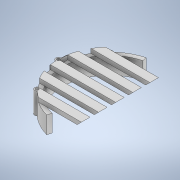
# Autodesk Inventor part: RoofNewShooterCup
Saved by Autodesk Inventor 2020 (Build 240168000, 168)
## iProperties
Created: 2021-04-22
Part Number: RoofNewShooterCup
Material: Generic
Document SubType Name: Modeling
Designer: tdmp4
Density: 1 g/cm^3
Appearance: Default
Author: tdmp4
Autodesk Inventor part; units mm, degrees
ref_plane "YZ Plane" through (0, 0, 0) normal (1, 0, 0) x (0, 1, 0)
ref_plane "XZ Plane" through (0, 0, 0) normal (0, 1, 0) x (-1, 0, 0)
ref_plane "XY Plane" through (0, 0, 0) normal (0, 0, 1) x (1, 0, 0)
sketch "Sketch1" plane through (0, 0, 0) normal (0, 1, 0) x (-1, 0, 0)
  circle A0 centre (0, 0) radius 72.39
  circle A1 centre (0, 0) radius 76.2
  circle A2 centre (76.2, 0) radius 3.81
  circle A3 centre (76.2, 0) radius 2.286
  circle A4 centre (0, 0) radius 69.85
  line L0 (0, 0) -> (53.8815, -53.8815)
  line L1 (0, 0) -> (76.2, 0) construction
  line L2 (0, 0) -> (53.8815, 53.8815)
  line L3 (0, 0) -> (76.2, 0) construction
  circle A5 centre (53.8815, 53.8815) radius 3.81
  circle A6 centre (53.8815, -53.8815) radius 3.81
  circle A7 centre (53.8815, -53.8815) radius 2.286
  circle A8 centre (53.8815, 53.8815) radius 2.286
  line L4 (0, 0) -> (18.0785, 67.4699)
  line L5 (0, 0) -> (69.85, 0) construction
  line L6 (18.0785, 67.4699) -> (19.722, 73.6035)
  line L7 (0, 0) -> (19.722, -73.6035)
  line L8 (0, 0) -> (76.2, 0) construction
  point P0 (76.1048, 3.8088)
  point P1 (56.5074, 51.1209)
  point P2 (51.1875, 51.1875)
  point P3 (49.3914, 49.3914)
  point P4 (49.3914, -49.3914)
  point P5 (51.1875, -51.1875)
  point P6 (56.5074, -51.1209)
  point P7 (76.1048, -3.8088)
  point P8 (51.1209, -56.5074)
  point P9 (18.0785, -67.4699)
  point P10 (51.1209, 56.5074)
  dimension "d4" = 139.7
  dimension "d0" = 144.78
  dimension "d1" = 152.4
  dimension "d2" = 7.62
  dimension "d3" = 4.572
  dimension "d5" = 45
  dimension "d6" = 45
  dimension "d7" = 4.572
  dimension "d8" = 4.572
  dimension "d11" = 75
  dimension "d12" = 75
  constraints: 18 end point, 8 centre point, 8 coincident, 5 point on circle, 4 equal length, 4 horizontal, 1 tangent, 3 other
  measures "d0" diameter of A0
  measures "d1" diameter of A1
  measures "d2" diameter of A2
  measures "d3" diameter of A3
  measures "d5" angle of L0 L1
  measures "d6" angle of L3 L2
  measures "d7" diameter of A7
  measures "d8" diameter of A8
  measures "d11" angle of L5 L4
  measures "d12" angle of L7 L8
extrude "Extrusion1" add sketch "Sketch1" along normal blind 25.4 contours A0 L0 A4 L2 | A2 A1 A6 A0 | A0 A5 A1 A2 | A2 A1 A3 | L2 A4 L6 A0 | A5 A1 A8 L2 | A0 L6 A1 A5 | L2 A8 A1 A5 | A6 A1 L7 A0 | A0 L7 A4 L0 | A6 A1 A7 L0 | L0 A7 A1 A6 | A2 A1 A3 | A5 A1 A8 | A6 A1 A7
sketch "Sketch2" plane through (0, 25.4, 0) normal (0, 1, 0) x (1, 0, 0)
  arc A0 (-76.1048, 3.8088) -> (-76.1048, -3.8088) centre (-76.2, 0) ccw projected
  line L0 (-80.01, 0) -> (-80.01, -76.2)
  line L1 (-80.01, -76.2) -> (-80.01, 76.2)
  line L2 (-80.01, 76.2) -> (21.59, 76.2) construction
  line L3 (-74.93, 63.5) -> (-74.93, 50.8)
  line L4 (-74.93, 50.8) -> (21.59, 50.8)
  line L5 (21.59, 50.8) -> (21.59, 38.1)
  line L6 (21.59, 38.1) -> (-74.93, 38.1)
  line L7 (-74.93, 38.1) -> (-74.93, 25.4)
  line L8 (-74.93, 25.4) -> (21.59, 25.4)
  line L9 (21.59, 25.4) -> (21.59, 12.7)
  line L10 (21.59, 12.7) -> (-74.93, 12.7)
  line L11 (-74.93, 12.7) -> (-74.93, 0)
  line L12 (-74.93, 0) -> (21.59, 0)
  line L13 (21.59, 0) -> (21.59, -12.7)
  line L14 (21.59, -12.7) -> (-74.93, -12.7)
  line L15 (-74.93, -12.7) -> (-74.93, -25.4)
  line L16 (-74.93, -25.4) -> (21.59, -25.4)
  line L17 (21.59, -25.4) -> (21.59, -38.1)
  line L18 (21.59, -38.1) -> (-74.93, -38.1)
  line L19 (-74.93, -38.1) -> (-74.93, -50.8)
  line L20 (-74.93, -50.8) -> (21.59, -50.8)
  line L21 (21.59, -50.8) -> (21.59, -63.5)
  line L22 (21.59, -63.5) -> (-75.5152, -63.5)
  line L23 (-75.5152, -63.5) -> (-75.5152, -76.2)
  line L24 (-75.5152, -76.2) -> (-80.01, -76.2)
  line L25 (-74.93, 63.5) -> (-74.93, 76.2)
  line L26 (-74.93, 63.5) -> (-80.01, 63.5)
  line L27 (-74.93, 50.8) -> (-80.01, 50.8)
  line L28 (-75.5152, -63.5) -> (-80.01, -63.5)
  circle A1 centre (-53.8815, -53.8815) radius 2.286 projected
  circle A2 centre (-53.8815, -53.8815) radius 2.286
  circle A3 centre (-53.8815, 53.8815) radius 2.286 projected
  circle A4 centre (-53.8815, 53.8815) radius 2.286
  circle A5 centre (-76.2, 0) radius 2.286 projected
  circle A6 centre (-76.2, 0) radius 2.286
  line L29 (-75.5152, -63.5) -> (-80.01, -63.5)
  point P0 (0, 0)
  point P1 (-73.914, 0)
  point P2 (-74.93, 1.9008)
  dimension "d13" = 76.2
  dimension "d14" = 152.4
  dimension "d20" = 12.7
  dimension "d21" = 12.7
  dimension "d22" = 12.7
  dimension "d23" = 12.7
  dimension "d24" = 96.52
  dimension "d25" = 90
  dimension "d26" = 12.7
  dimension "d27" = 12.7
  dimension "d28" = 96.52
  dimension "d29" = 90
  dimension "d30" = 12.7
  dimension "d31" = 12.7
  dimension "d32" = 90
  dimension "d33" = 12.7
  dimension "d34" = 12.7
  constraints: 60 end point, 19 point on line, 11 perpendicular, 5 horizontal, 3 centre point, 3 coincident, 1 point on circle, 1 tangent, 1 vertical
  measures "d13" distance of L0.start L0.end
  measures "d14" distance of L0.end L1.end
  measures "d20" distance of L3.start L3.end
  measures "d21" distance of L4.end L5.end
  measures "d22" distance of L6.end L7.end
  measures "d23" distance of L8.end L9.end
  measures "d24" distance of L9.end L10.end
  measures "d25" angle of L9 L10
  measures "d26" distance of L10.end L11.end
  measures "d27" distance of L12.end L13.end
  measures "d28" distance of L13.end L14.end
  measures "d29" angle of L13 L14
  measures "d30" distance of L14.end L15.end
  measures "d31" distance of L16.end L17.end
  measures "d32" angle of L17 L18
  measures "d33" distance of L18.end L19.end
  measures "d34" distance of L20.end L21.end
extrude "Extrusion2" add sketch "Sketch2" along normal blind 6.35 contours L1 L27 L4 L5 L6 L7 L8 L9 L10 L11 A5 L12 L13 L14 L15 L16 L17 L18 L19 L20 L21 L22 L28 L0
sketch "Sketch3" plane through (0, 31.75, 0) normal (0, 1, 0) x (1, 0, 0)
  arc A0 (-19.722, 73.6035) -> (-51.1209, 56.5074) centre (0, 0) ccw projected
  line L0 (-29.0994, -63.5) -> (-42.1211, -63.5) projected
  arc A1 (-41.3516, 64.0038) -> (-42.1211, -63.5) centre (0, 0) ccw
  circle A2 centre (-76.2, 0) radius 3.81
  line L1 (-80.01, -63.5) -> (-42.1211, -63.5) projected
  line L2 (-42.1211, -63.5) -> (-144.5648, -63.5)
  line L3 (-144.5648, -63.5) -> (-144.5648, 70.3259)
  line L4 (-144.5648, 70.3259) -> (-41.3516, 64.0038)
  circle A3 centre (-53.8815, -53.8815) radius 2.286 projected
  circle A4 centre (-53.8815, -53.8815) radius 3.81
  point P0 (-51.1209, -56.5074)
  point P1 (-56.5074, -51.1209)
  point P2 (-76.1048, -3.8088)
  point P3 (-76.1048, 3.8088)
  point P4 (-51.1209, 56.5074)
  dimension "d37" = 7.62
  dimension "d38" = 7.62
  constraints: 6 end point, 4 point on circle, 3 centre point, 1 coincident, 1 concentric, 1 horizontal, 1 perpendicular
  measures "d37" diameter of A2
  measures "d38" diameter of A4
extrude "Extrusion3" cut sketch "Sketch3" against normal blind 6.35 contours A0 A1 A2 A4 L1 L2 L3 L4
chamfer "Chamfer1" distance 6.35 angle 45 5 edges at (21.59, 25.4, 57.15) (21.59, 25.4, 31.75) (21.59, 25.4, 6.35) (21.59, 25.4, -19.05) (21.59, 25.4, -44.45)
body "Solid1"
